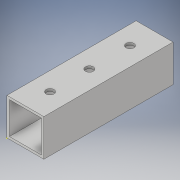
# Autodesk Inventor part: 足2
Saved by Autodesk Inventor 2019 (Build 230136000, 136)
## iProperties
Created: 2022-04-06
Part Number: 足2
Material: 一般
Document SubType Name: Sheet Metal
Designer: yuta
Density: 1 g/cm^3
Sheet Metal Rule: Default_mm
Appearance: 既定
Author: yuta
Autodesk Inventor part; units mm, degrees
ref_plane "YZ Plane" through (0, 0, 0) normal (1, 0, 0) x (0, 1, 0)
ref_plane "XZ Plane" through (0, 0, 0) normal (0, 1, 0) x (-1, 0, 0)
ref_plane "XY Plane" through (0, 0, 0) normal (0, 0, 1) x (1, 0, 0)
sketch "スケッチ1" plane through (0, 0, 0) normal (0, 0, 1) x (1, 0, 0)
  line L0 (0, 0) -> (15, 0)
  line L1 (15, 0) -> (15, 15)
  line L2 (15, 15) -> (0, 15)
  line L3 (0, 15) -> (0, 0)
  dimension "d0" = 15
  dimension "d1" = 15
  constraints: 8 end point, 2 parallel, 1 horizontal, 1 perpendicular
  measures "d0" distance of L2.end L1.end
  measures "d1" distance of L1.end L0.end
extrude "押し出し1" add sketch "スケッチ1" along normal blind 52.5
sketch "スケッチ2" plane through (0, 0, 52.5) normal (0, 0, 1) x (1, 0, 0)
  point P0 (0, 0)
sketch "スケッチ3" plane through (0, 0, 52.5) normal (0, 0, 1) x (1, 0, 0)
  line L0 (1, 1) -> (14, 1)
  line L1 (14, 1) -> (14, 14)
  line L2 (14, 14) -> (1, 14)
  line L3 (1, 14) -> (1, 1)
  line L4 (15, 15) -> (0, 15) projected
  line L5 (15, 0) -> (15, 15) projected
  point P0 (0, 0)
  dimension "d4" = 13
  dimension "d5" = 13
  dimension "d6" = 1
  dimension "d7" = 1
  constraints: 8 end point, 2 parallel, 1 horizontal, 1 perpendicular
  measures "d4" distance of L2.end L1.end
  measures "d5" distance of L1.end L0.end
  measures "d6" distance between parallel lines of L4 L2
  measures "d7" distance between parallel lines of L5 L1
extrude "押し出し2" cut sketch "スケッチ3" against normal blind 52.5
sketch "スケッチ4" plane through (0, 15, 0) normal (0, 1, 0) x (1, 0, 0)
  circle A0 centre (7.5, -42.5) radius 1.6
  line L0 (15, -52.5) -> (0, -52.5) projected
  line L1 (15, 0) -> (15, -52.5) projected
  circle A1 centre (7.5, -10) radius 1.6
  line L2 (15, 0) -> (0, 0) projected
  circle A2 centre (7.5, -26.5) radius 1.6
  dimension "d10" = 3.2
  dimension "d11" = 10
  dimension "d12" = 7.5
  dimension "d13" = 3.2
  dimension "d14" = 10
  dimension "d15" = 7.5
  dimension "d16" = 3.2
  dimension "d17" = 16
  dimension "d18" = 16.5
  constraints: 3 centre point
  measures "d10" diameter of A0
  measures "d11" distance from line of L0 A0.centre
  measures "d12" distance from line of L1 A0.centre
  measures "d13" diameter of A1
  measures "d14" distance from line of L2 A1.centre
  measures "d15" distance from line of L1 A1.centre
  measures "d16" diameter of A2
  measures "d17" distance of A2.centre A0.centre
  measures "d18" distance of A1.centre A2.centre
hole "穴1" at (7.5, 15, 26.5) at (7.5, 15, 10) at (7.5, 15, 42.5) direction (0, -1, 0) diameter 3.2 depth 15
equation "\"BendRadius\" = Thickness"
equation "\"BendReliefWidth\" = Thickness"
equation "\"BendReliefDepth\" = 0.5 * Thickness"
equation "\"CornerReliefSize\" = 4 * Thickness"
equation "\"MinimumRemnant\" = 2 * Thickness"
equation "\"TransitionRadius\" = BendRadius"
equation "\"JacobiRadiusSize\" = BendRadius"
equation "\"GapSize\" = Thickness"
equation "\"Thickness\" = 0.5"
